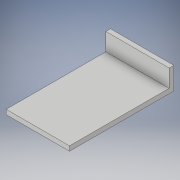
# Autodesk Inventor part: Platinenhalter-einzeln
Saved by Autodesk Inventor 2017.3 (Build 213256000, 256)
## iProperties
Part Number: Platinenhalter-einzeln
Material: Generisch
Document SubType Name: Modeling
Designer: Nils
Density: 1 g/cm^3
Appearance: Vorgabe
Author: Nils
Autodesk Inventor part; units mm, degrees
ref_plane "YZ Plane" through (0, 0, 0) normal (1, 0, 0) x (0, 1, 0)
ref_plane "XZ Plane" through (0, 0, 0) normal (0, 1, 0) x (-1, 0, 0)
ref_plane "XY Plane" through (0, 0, 0) normal (0, 0, 1) x (1, 0, 0)
sketch "Skizze1" plane through (0, 0, 0) normal (1, 0, 0) x (0, 1, 0)
  line L0 (-44.5, -5.5) -> (40.5, -5.5)
  line L1 (44.5, -9.5) -> (-44.5, -9.5)
  line L2 (-44.5, -9.5) -> (-44.5, -5.5)
  line L3 (40.5, -5.5) -> (40.5, 9.5)
  line L4 (40.5, 9.5) -> (44.5, 9.5)
  line L5 (44.5, 9.5) -> (44.5, -9.5)
  point P0 (0, 0)
  point P1 (44.5, 0)
  point P2 (0, -9.5)
  dimension "d0" = 4
  dimension "d2" = 4
  dimension "d3" = 19
  dimension "d6" = 89
  constraints: 12 end point, 2 horizontal, 2 midpoint, 2 parallel, 2 vertical, 1 horizontal alignment, 1 vertical alignment
  measures "d0" distance of L1.end L0.start
  measures "d2" distance of L3.end L4.end
  measures "d3" distance of L4.end L1.start
  measures "d6" distance of L1.start L1.end
extrude "Extrusion1" add sketch "Skizze1" along normal mid plane 54
